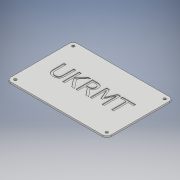
# Autodesk Inventor part: TestingRemoteBackplate
Saved by Autodesk Inventor 2018.3 (Build 223284000, 284)
## iProperties
Created: 2019-03-25
Part Number: TestingRemoteBackplate
Material: Generic
Document SubType Name: Modeling
Designer: matth
Density: 1 g/cm^3
Appearance: Default
Author: matth
Autodesk Inventor part; units mm, degrees
note: some values were not read from the file. Chosen so that the rebuilt part matches the saved one: direction of "Emboss1".
ref_plane "YZ Plane" through (0, 0, 0) normal (1, 0, 0) x (0, 1, 0)
ref_plane "XZ Plane" through (0, 0, 0) normal (0, 1, 0) x (-1, 0, 0)
ref_plane "XY Plane" through (0, 0, 0) normal (0, 0, 1) x (1, 0, 0)
sketch "Sketch1" plane through (0, 0, 0) normal (0, 0, 1) x (1, 0, 0)
  line L0 (-6.4379, 104.6218) -> (131.9621, 104.6218)
  line L1 (138.9621, 97.6218) -> (138.9621, 10.0218)
  line L2 (131.9621, 3.0218) -> (-6.4379, 3.0218)
  line L3 (-13.4379, 10.0218) -> (-13.4379, 97.6218)
  arc A0 (-13.4379, 10.0218) -> (-6.4379, 3.0218) centre (-6.4379, 10.0218) ccw
  arc A1 (-6.4379, 104.6218) -> (-13.4379, 97.6218) centre (-6.4379, 97.6218) ccw
  arc A2 (138.9621, 97.6218) -> (131.9621, 104.6218) centre (131.9621, 97.6218) ccw
  arc A3 (131.9621, 3.0218) -> (138.9621, 10.0218) centre (131.9621, 10.0218) ccw
  circle A4 centre (-6.4379, 97.6218) radius 2
  circle A5 centre (131.9621, 97.6218) radius 2
  circle A6 centre (131.9621, 10.0218) radius 2
  circle A7 centre (-6.4379, 10.0218) radius 2
  point P0 (0, 0)
  point P1 (-13.4379, 104.6218)
  point P2 (138.9621, 3.0218)
  point P3 (-13.4379, 3.0218)
  dimension "d0" = 152.4
  dimension "d1" = 101.6
  dimension "d2" = 7
  dimension "d3" = 4
  dimension "d4" = 4
  dimension "d5" = 4
  dimension "d6" = 4
  constraints: 8 centre point, 8 end point, 8 point on circle, 8 tangent, 6 point on line, 4 coincident, 3 equal radius, 2 parallel, 1 horizontal, 1 perpendicular
  measures "d0" distance of point (138.962, 3.022) point (-13.438, 3.022)
  measures "d1" distance of point (-13.438, 3.022) point (-13.438, 104.622)
  measures "d2" radius of A0
  measures "d3" diameter of A4
  measures "d4" diameter of A5
  measures "d5" diameter of A6
  measures "d6" diameter of A7
extrude "Extrusion1" add sketch "Sketch1" along normal blind 2
chamfer "Chamfer1" distance 0.5 distance2 2 8 edges at (62.7621, 3.0218, 2) (136.9118, 5.072, 2) (138.9621, 53.8218, 2) (136.9118, 102.5715, 2) (62.7621, 104.6218, 2) (-11.3877, 102.5715, 2) (-13.4379, 53.8218, 2) (-11.3877, 5.072, 2) measured on face at (40.2857, 68.1119, 2)
sketch "Sketch2" plane through (0, 0, 2) normal (0, 0, 1) x (1, 0, 0)
  line L0 (6.8688, 68.1594) -> (119.5871, 68.1594) construction
  line L1 (119.5871, 68.1594) -> (119.5871, -3.3463) construction
  line L2 (119.5871, -3.3463) -> (6.8688, -3.3463) construction
  line L3 (6.8688, -3.3463) -> (6.8688, 68.1594) construction
  spline S0 degree 2 poles (18.133, 42.6326) (15.9247, 42.6326) (12.6427, 43.7874) (11.4879, 44.9422) knots 0 0 0 1 2 2 2
  spline S1 degree 2 poles (11.4879, 44.9422) (10.171, 46.2388) (9.0973, 49.8855) (9.0973, 52.5597) knots 0 0 0 1 2 2 2
  line L4 (9.0973, 52.5597) -> (9.0973, 68.1594)
  line L5 (9.0973, 68.1594) -> (12.4198, 68.1594)
  line L6 (12.4198, 68.1594) -> (12.4198, 52.5597)
  spline S2 degree 2 poles (12.4198, 52.5597) (12.4198, 50.8174) (12.8655, 48.4673) (13.4936, 47.5151) knots 0 0 0 1 2 2 2
  spline S3 degree 2 poles (13.4936, 47.5151) (14.1621, 46.5022) (16.4717, 45.469) (18.133, 45.469) knots 0 0 0 1 2 2 2
  spline S4 degree 2 poles (18.133, 45.469) (19.6929, 45.469) (22.124, 46.5022) (22.7926, 47.5151) knots 0 0 0 1 2 2 2
  spline S5 degree 2 poles (22.7926, 47.5151) (23.4206, 48.4673) (23.8663, 50.7972) (23.8663, 52.4787) knots 0 0 0 1 2 2 2
  line L7 (23.8663, 52.4787) -> (23.8663, 68.1594)
  line L8 (23.8663, 68.1594) -> (27.1889, 68.1594)
  line L9 (27.1889, 68.1594) -> (27.1889, 52.5597)
  spline S6 degree 2 poles (27.1889, 52.5597) (27.1889, 49.9463) (26.1354, 46.2185) (24.7983, 44.9422) knots 0 0 0 1 2 2 2
  spline S7 degree 2 poles (24.7983, 44.9422) (23.603, 43.7672) (20.4425, 42.6326) (18.133, 42.6326) knots 0 0 0 1 2 2 2
  line L10 (50.1832, 43.1594) -> (45.868, 43.1594)
  line L11 (45.868, 43.1594) -> (36.731, 54.7882)
  line L12 (36.731, 54.7882) -> (35.2723, 53.1472)
  line L13 (35.2723, 53.1472) -> (35.2723, 43.1594)
  line L14 (35.2723, 43.1594) -> (31.9498, 43.1594)
  line L15 (31.9498, 43.1594) -> (31.9498, 68.1594)
  line L16 (31.9498, 68.1594) -> (35.2723, 68.1594)
  line L17 (35.2723, 68.1594) -> (35.2723, 56.6724)
  line L18 (35.2723, 56.6724) -> (45.5236, 68.1594)
  line L19 (45.5236, 68.1594) -> (49.5754, 68.1594)
  line L20 (49.5754, 68.1594) -> (39.2229, 56.9965)
  line L21 (39.2229, 56.9965) -> (50.1832, 43.1594)
  line L22 (71.5163, 43.1594) -> (67.201, 43.1594)
  line L23 (67.201, 43.1594) -> (59.2999, 53.1067)
  line L24 (59.2999, 53.1067) -> (55.4911, 53.1067)
  line L25 (55.4911, 53.1067) -> (55.4911, 43.1594)
  line L26 (55.4911, 43.1594) -> (52.1686, 43.1594)
  line L27 (52.1686, 43.1594) -> (52.1686, 68.1594)
  line L28 (52.1686, 68.1594) -> (58.6111, 68.1594)
  spline S8 degree 2 poles (58.6111, 68.1594) (60.7586, 68.1594) (63.6556, 67.6934) (64.9725, 66.8425) knots 0 0 0 1 2 2 2
  spline S9 degree 2 poles (64.9725, 66.8425) (66.2894, 65.9916) (67.8088, 63.3377) (67.8088, 61.3725) knots 0 0 0 1 2 2 2
  spline S10 degree 2 poles (67.8088, 61.3725) (67.8088, 58.6375) (65.013, 54.9301) (62.6224, 54.0386) knots 0 0 0 1 2 2 2
  line L29 (62.6224, 54.0386) -> (71.5163, 43.1594)
  spline S11 degree 2 poles (64.3445, 61.1091) (64.3445, 62.2031) (63.5746, 63.8847) (62.7642, 64.4317) knots 0 0 0 1 2 2 2
  spline S12 degree 2 poles (62.7642, 64.4317) (62.0552, 64.8976) (60.171, 65.2826) (58.7934, 65.2826) knots 0 0 0 1 2 2 2
  line L30 (58.7934, 65.2826) -> (55.4911, 65.2826)
  line L31 (55.4911, 65.2826) -> (55.4911, 55.8822)
  line L32 (55.4911, 55.8822) -> (58.4085, 55.8822)
  spline S13 degree 2 poles (58.4085, 55.8822) (59.8469, 55.8822) (62.1362, 56.3887) (62.9263, 57.1788) knots 0 0 0 1 2 2 2
  spline S14 degree 2 poles (62.9263, 57.1788) (63.6556, 57.8677) (64.3445, 59.8125) (64.3445, 61.1091) knots 0 0 0 1 2 2 2
  line L33 (94.936, 43.1594) -> (91.6135, 43.1594)
  line L34 (91.6135, 43.1594) -> (91.6135, 64.695)
  line L35 (91.6135, 64.695) -> (85.09, 50.0476)
  line L36 (85.09, 50.0476) -> (83.0641, 50.0476)
  line L37 (83.0641, 50.0476) -> (76.6014, 64.695)
  line L38 (76.6014, 64.695) -> (76.6014, 43.1594)
  line L39 (76.6014, 43.1594) -> (73.5017, 43.1594)
  line L40 (73.5017, 43.1594) -> (73.5017, 68.1594)
  line L41 (73.5017, 68.1594) -> (78.0398, 68.1594)
  line L42 (78.0398, 68.1594) -> (84.2796, 54.2412)
  line L43 (84.2796, 54.2412) -> (90.3169, 68.1594)
  line L44 (90.3169, 68.1594) -> (94.936, 68.1594)
  line L45 (94.936, 68.1594) -> (94.936, 43.1594)
  line L46 (105.8355, 43.1594) -> (105.8355, 65.2015)
  line L47 (105.8355, 65.2015) -> (97.4482, 65.2015)
  line L48 (97.4482, 65.2015) -> (97.4482, 68.1594)
  line L49 (97.4482, 68.1594) -> (117.5454, 68.1594)
  line L50 (117.5454, 68.1594) -> (117.5454, 65.2015)
  line L51 (117.5454, 65.2015) -> (109.1581, 65.2015)
  line L52 (109.1581, 65.2015) -> (109.1581, 43.1594)
  line L53 (109.1581, 43.1594) -> (105.8355, 43.1594)
  point P0 (0, 0)
  constraints: 2 other
emboss "Emboss1" sketch "Sketch2" operation cut depth 1 direction (0, 0, -1)
body "Solid1"
